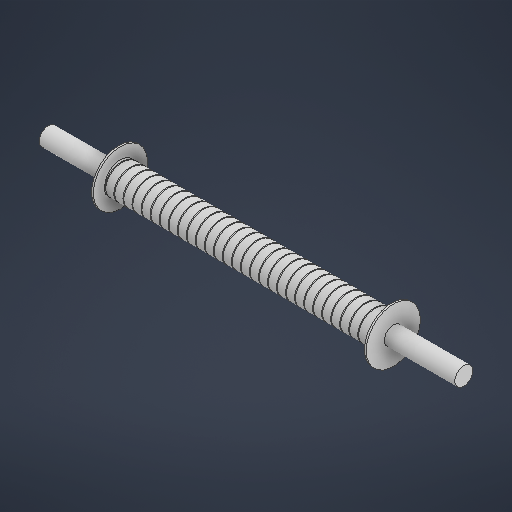
# Autodesk Inventor part: cam shaft
Saved by Autodesk Inventor 2026.1 (Build 301233020, 233B)
## iProperties
Created: 2025-12-31
Part Number: cam shaft
Material: Generic
Document SubType Name: Modeling
Designer: Austin Ngobeni
Density: 1 g/cm^3
Appearance: Default
Author: Austin Ngobeni
Autodesk Inventor part; units mm, degrees
ref_plane "YZ Plane" through (0, 0, 0) normal (1, 0, 0) x (0, 1, 0)
ref_plane "XY Plane" through (0, 0, 0) normal (0, 0, 1) x (1, 0, 0)
sketch "Sketch1" plane through (0, 0, 0) normal (1, 0, 0) x (0, 1, 0)
  circle A0 centre (0, 0) radius 17.5
  circle A1 centre (0, 0) radius 30
  dimension "d1" = 35
  dimension "d9" = 60
  constraints: 2 centre point, 1 coincident
  measures "d1" diameter of A0
  measures "d9" diameter of A1
extrude "Extrusion2" add sketch "Sketch1" along normal blind 300 contours A0
sketch "Sketch2" plane through (0, 0, 0) normal (-1, 0, 0) x (0, 0, 1)
  circle A0 centre (0, 0) radius 10
  dimension "d6" = 20
  constraints: 1 centre point, 1 coincident
  measures "d6" diameter of A0
extrude "Extrusion3" add sketch "Sketch2" along normal blind 80
extrude "Extrusion4" add sketch "Sketch1" against normal blind 2 contours A0 | A1
sketch "Sketch3" plane through (300, 0, 0) normal (1, 0, 0) x (0, 0, -1)
  circle A0 centre (0, 0) radius 30 projected
  circle A1 centre (0, 0) radius 10 projected
extrude "Extrusion5" add sketch "Sketch3" along normal blind 80 contours A1
extrude "Extrusion6" add sketch "Sketch3" along normal blind 2
sketch "Sketch4" plane through (300, 0, 0) normal (1, 0, 0) x (0, 0, -1)
  circle A0 centre (0, 0) radius 17.5 projected
ref_plane "Work Plane3" through (300, -8.1347, 15.4944) normal (0, 1, 0) x (-1, 0, 0)
sketch "Sketch8" plane through (300, -8.1347, 15.4944) normal (0, 1, 0) x (-1, 0, 0)
  circle A0 centre (0, 0) radius 0.5
  point P0 (300, -15.4944)
  dimension "d47" = 1
  constraints: 1 centre point
  measures "d47" diameter of A0
sketch3d "3D Sketch3"
  helix H0 starts at (300, -8.1347, 15.4944) axis through (300, 0, 0) along (-1, 0, 0) pitch 10 turns 30 hand left
sweep "Sweep1" cut profiles "Sketch8" path "3D Sketch3"
sweep "Sweep2" [suppressed]
body "Solid1"
